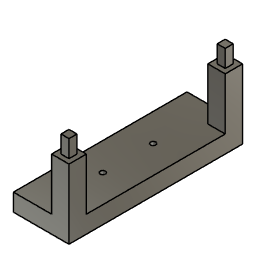
WRO Back v2 (1) (Autodesk Fusion 360 design; units mm, degrees)
Autodesk Fusion 360 part; units mm, degrees
note: some values were not read from the file. Set by a fixed rule: which sketch regions a step uses.
sketch "Sketch1" plane through (0, 0, 0) normal (0, 0, 1) x (1, 0, 0)
sketch "Sketch2" plane through (0, 0, 0) normal (0, 1, 0) x (1, 0, 0)
  line L0 (0, 0) -> (-16, 0)
  line L1 (-16, 0) -> (-16, -5)
  line L2 (-16, -5) -> (0, -5)
  line L3 (0, -5) -> (0, 0)
  line L4 (0, 0) -> (-5, 0)
  line L5 (-5, 0) -> (-5, -25)
  line L6 (-5, -25) -> (0, -25)
  line L7 (0, -25) -> (0, 0)
  dimension "d1" = 16
  dimension "d2" = 5
  dimension "d3" = 5
  dimension "d4" = 25
  constraint horizontal L0
  constraint vertical L1
  constraint horizontal L2
  constraint vertical L3
  constraint coincident L0.start L3.end
  constraint horizontal L4
  constraint vertical L5
  constraint horizontal L6
  constraint vertical L7
  measures "d1" distance of L0.start L0.end
  measures "d2" distance of L0.start L2.end
  measures "d3" distance of L0.start L4.end
  measures "d4" distance of L0.start L6.end
extrude "Extrude1" add sketch "Sketch2" along normal blind 50
sketch "Sketch3" plane through (-5, 0, 0) normal (-1, 0, 0) x (0, -1, 0)
  line L0 (0, 5) -> (0, 25)
  line L1 (0, 25) -> (-50, 25)
  line L2 (-50, 25) -> (-50, 5)
  line L3 (-50, 5) -> (0, 5)
  line L4 (-50, 5) -> (-45, 5)
  line L5 (-45, 5) -> (-5, 5)
  line L6 (-5, 5) -> (-5, 20)
  line L7 (-5, 20) -> (-45, 20)
  line L8 (-45, 20) -> (-45, 5)
  dimension "d7" = 5
  dimension "d8" = 40
  dimension "d9" = 15
  constraint coincident L2.end L3.start
  constraint perpendicular L2 L4
  constraint horizontal L5
  constraint vertical L6
  constraint horizontal L7
  constraint vertical L8
  measures "d7" distance of L2.end L4.end
  measures "d8" distance of L4.end L5.end
  measures "d9" distance of L4.end L7.end
extrude "Extrude2" cut sketch "Sketch3" against normal blind 1000 contours L3 L5 L6 L7 L8
sketch "Sketch4" plane through (0, 0, 25) normal (0, 0, 1) x (-1, 0, 0)
  line L0 (5, 0) -> (0, 0)
  line L1 (0, 0) -> (0, -50)
  line L2 (0, -50) -> (5, -50)
  line L3 (5, -50) -> (5, 0)
  line L4 (0, -50) -> (0, -48.675)
  line L5 (0, -48.675) -> (1.325, -48.675)
  line L6 (1.325, -48.675) -> (3.625, -48.675)
  line L7 (3.625, -48.675) -> (3.625, -46.375)
  line L8 (3.625, -46.375) -> (1.325, -46.375)
  line L9 (1.325, -46.375) -> (1.325, -48.675)
  line L10 (0, 0) -> (0, -1.325)
  line L11 (0, -1.325) -> (1.325, -1.325)
  line L12 (1.325, -1.325) -> (3.625, -1.325)
  line L13 (3.625, -1.325) -> (3.625, -3.625)
  line L14 (3.625, -3.625) -> (1.325, -3.625)
  line L15 (1.325, -3.625) -> (1.325, -1.325)
  dimension "d12" = 1.325
  dimension "d13" = 1.325
  dimension "d14" = 2.3
  dimension "d15" = 2.3
  dimension "d16" = 1.325
  dimension "d17" = 1.325
  dimension "d18" = 2.3
  dimension "d19" = 2.3
  constraint coincident L1.end L2.start
  constraint perpendicular L2 L4
  constraint perpendicular L4 L5
  constraint horizontal L6
  constraint vertical L7
  constraint horizontal L8
  constraint vertical L9
  constraint coincident L0.end L1.start
  constraint perpendicular L0 L10
  constraint perpendicular L10 L11
  constraint horizontal L12
  constraint vertical L13
  constraint horizontal L14
  constraint vertical L15
  measures "d12" distance of L1.end L4.end
  measures "d13" distance of L4.end L5.end
  measures "d14" distance of L5.end L6.end
  measures "d15" distance of L5.end L8.end
  measures "d16" distance of L0.end L10.end
  measures "d17" distance of L10.end L11.end
  measures "d18" distance of L11.end L12.end
  measures "d19" distance of L11.end L14.end
extrude "Extrude3" cut sketch "Sketch4" against normal blind 5
sketch "Sketch5" plane through (0, 0, 5) normal (0, 0, 1) x (-1, 0, 0)
  line L0 (16, 0) -> (5, 0)
  line L1 (5, 0) -> (5, -5)
  line L2 (5, -5) -> (0, -5)
  line L3 (0, -5) -> (0, -45)
  line L4 (0, -45) -> (5, -45)
  line L5 (5, -45) -> (5, -50)
  line L6 (5, -50) -> (16, -50)
  line L7 (16, -50) -> (16, 0)
  line L8 (8, -50) -> (8, -25)
  line L9 (8, -25) -> (8, -32.25)
  line L10 (8, -32.25) -> (8, -17.75)
  line L11 (0, -36) -> (7.25, -36)
  line L12 (7.25, -36) -> (7.25, -31.1746)
  line L13 (8, -32.25) -> (7.25, -32.25)
  line L14 (7.25, -32.25) -> (8, -32.25)
  circle A0 centre (8, -32.25) radius 0.75
  line L15 (8, -32.25) -> (8, -17.75)
  circle A1 centre (8, -17.75) radius 0.75
  dimension "d22" = 25
  dimension "d23" = 7.25
  dimension "d24" = 14.5
  dimension "d25" = 7.25
  dimension "d26" = 0.75
  dimension "d27" = 1.5
  dimension "d28" = 14.5
  dimension "d29" = 1.5
  constraint coincident L6 L8.start
  constraint perpendicular L0 L8
  constraint parallel L8 L9
  constraint parallel L8 L10
  constraint coincident L3 L11.start
  constraint perpendicular L3 L11
  constraint perpendicular L11 L12
  constraint coincident L12 L13.end
  constraint perpendicular L12 L13
  constraint perpendicular L12 L14
  constraint coincident L9.end L10.start
  constraint parallel L10 L15
  constraint coincident L10.end L15.end
  measures "d22" distance of L8.start L8.end
  measures "d23" distance of L8.end L9.end
  measures "d24" distance of L9.end L10.end
  measures "d25" distance of L11.start L11.end
  measures "d26" distance of L13.end L9.end
  measures "d27" diameter of A0
  measures "d28" distance of L9.end L10.end
  measures "d29" diameter of A1
extrude "Extrude4" cut sketch "Sketch5" against normal blind 1000 contours L8 L13 L14 A0 | L8 L9 L10 A0 L15 | L8 L9 L10 L13 L14 A0 L15 | A1
extrude "Extrude5" cut 2 faces at (-2.8583, 47.1417, 25) (-2.0917, 2.8583, 25) along direction (0, 0, -1) blind 5
sketch "Sketch6" plane through (0, 0, 20) normal (0, 0, 1) x (-1, 0, 0)
  line L0 (5, -45) -> (0, -45)
  line L1 (0, -45) -> (0, -50)
  line L2 (0, -50) -> (5, -50)
  line L3 (5, -50) -> (5, -45)
  line L4 (5, 0) -> (3.65, 0)
  line L5 (3.65, 0) -> (3.65, -1.35)
  line L6 (3.65, -1.35) -> (5, -1.35)
  line L7 (5, -1.35) -> (5, 0)
  line L8 (3.65, -1.35) -> (1.35, -1.35)
  line L9 (1.35, -1.35) -> (1.35, -3.65)
  line L10 (1.35, -3.65) -> (3.65, -3.65)
  line L11 (3.65, -3.65) -> (3.65, -1.35)
  line L12 (5, -45) -> (3.65, -45)
  line L13 (3.65, -45) -> (3.65, -46.35)
  line L14 (3.65, -46.35) -> (5, -46.35)
  line L15 (5, -46.35) -> (5, -45)
  line L16 (3.65, -46.35) -> (1.35, -46.35)
  line L17 (1.35, -46.35) -> (1.35, -48.65)
  line L18 (1.35, -48.65) -> (3.65, -48.65)
  line L19 (3.65, -48.65) -> (3.65, -46.35)
  dimension "d34" = 1.35
  dimension "d35" = 1.35
  dimension "d36" = 2.3
  dimension "d37" = 2.3
  dimension "d38" = 1.35
  dimension "d39" = 1.35
  dimension "d40" = 2.3
  dimension "d41" = 2.3
  constraint horizontal L4
  constraint vertical L5
  constraint horizontal L6
  constraint vertical L7
  constraint horizontal L8
  constraint vertical L9
  constraint horizontal L10
  constraint vertical L11
  constraint horizontal L12
  constraint vertical L13
  constraint horizontal L14
  constraint vertical L15
  constraint coincident L0.start L3.end
  constraint horizontal L16
  constraint vertical L17
  constraint horizontal L18
  constraint vertical L19
  measures "d34" distance of L4.start L4.end
  measures "d35" distance of L4.start L6.end
  measures "d36" distance of L5.end L8.end
  measures "d37" distance of L5.end L10.end
  measures "d38" distance of L0.start L12.end
  measures "d39" distance of L0.start L14.end
  measures "d40" distance of L13.end L16.end
  measures "d41" distance of L13.end L18.end
extrude "Extrude6" add sketch "Sketch6" along normal blind 5 contours L16 L17 L18 L19 | L8 L9 L10 L11
